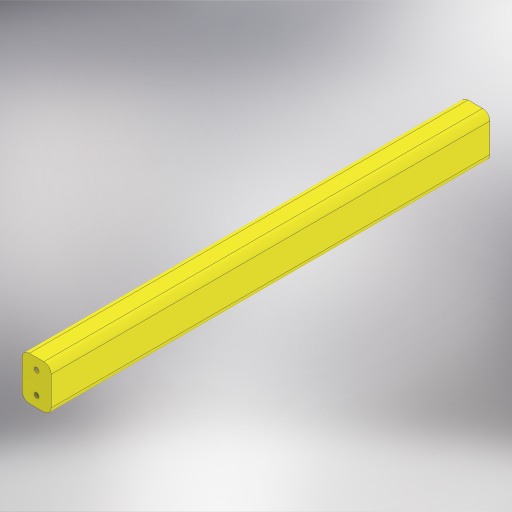
# Autodesk Inventor part: handle handle
Saved by Autodesk Inventor 2024 (Build 280153000, 153)
## iProperties
Created: 2023-01-06
Part Number: handle handle
Material: Generic
Document SubType Name: Modeling
Designer: Hayden Swanson
Density: 1 g/cm^3
Appearance: Default
Author: Hayden Swanson
Autodesk Inventor part; units mm, degrees
ref_plane "YZ Plane" through (0, 0, 0) normal (1, 0, 0) x (0, 1, 0)
ref_plane "XZ Plane" through (0, 0, 0) normal (0, 1, 0) x (-1, 0, 0)
ref_plane "XY Plane" through (0, 0, 0) normal (0, 0, 1) x (1, 0, 0)
sketch "Sketch1" plane through (0, 0, 0) normal (0, 0, 1) x (1, 0, 0)
  line L0 (0, 0) -> (12.7, 0)
  line L1 (12.7, 0) -> (12.7, 19.05)
  line L2 (12.7, 19.05) -> (0, 19.05)
  line L3 (0, 19.05) -> (0, 0)
  dimension "d0" = 12.7
  dimension "d1" = 19.05
  constraints: 8 end point, 2 parallel, 1 horizontal, 1 perpendicular
  measures "d0" distance of L2.end L1.end
  measures "d1" distance of L0.end L1.end
extrude "Extrusion1" add sketch "Sketch1" along normal blind 191.516
sketch "Sketch2" plane through (0, 0, 191.516) normal (0, 0, 1) x (1, 0, 0)
  line L0 (12.7, 19.05) -> (0, 19.05) projected
  line L1 (6.35, 19.05) -> (6.35, 0)
  line L2 (6.35, 19.05) -> (6.35, 9.525)
  circle A0 centre (6.35, 14.2875) radius 1.4224
  line L3 (6.35, 9.525) -> (6.35, 0)
  line L4 (0, 0) -> (12.7, 0) projected
  circle A1 centre (6.35, 4.7625) radius 1.4224
  dimension "d4" = 2.8448
  dimension "d5" = 2.8448
  constraints: 6 end point, 4 midpoint, 2 centre point, 1 perpendicular, 1 vertical
  measures "d4" diameter of A0
  measures "d5" diameter of A1
sketch "Sketch3" plane through (0, 0, 0) normal (0, 0, -1) x (-1, 0, 0)
  line L0 (-12.7, 19.05) -> (0, 19.05) projected
  line L1 (-6.35, 19.05) -> (-6.35, 0)
  circle A0 centre (-6.35, 14.2875) radius 1.4224 projected
  circle A1 centre (-6.35, 14.2875) radius 1.4224
  circle A2 centre (-6.35, 4.7625) radius 1.4224 projected
  circle A3 centre (-6.35, 4.7625) radius 1.4224
  point P0 (0, 0)
  constraints: 2 centre point, 2 coincident, 2 end point, 1 midpoint, 1 vertical
fillet "Fillet1" radius 3.175 4 edges at (12.7, 19.05, 95.758) (0, 19.05, 95.758) (0, 0, 95.758) (12.7, 0, 95.758)
hole "Hole1" at (6.35, 4.7625, 191.516) at (6.35, 14.2875, 191.516) direction (0, 0, -1) diameter 2.1565 depth 25.4 tip angle 118 thread size "4-40 UNC" class "3B" standard "ANSI Unified Screw Threads"
hole "Hole2" at (6.35, 4.7625, 0) at (6.35, 14.2875, 0) direction (0, 0, 1) diameter 2.1565 depth 25.4 tip angle 118 thread size "4-40 UNC" class "3B" standard "ANSI Unified Screw Threads"
body "Solid1"
